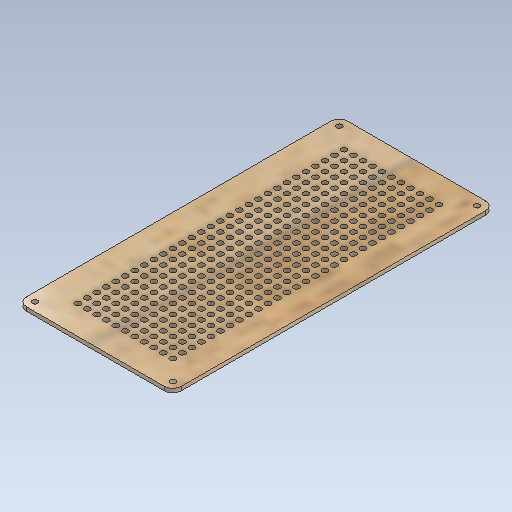
# Autodesk Inventor part: ロボット回転_回路ボード1
Saved by Autodesk Inventor 2020.3 (Build 243373000, 373)
## iProperties
Created: 2020-07-06
Part Number: ロボット回転_回路ボード1
Material: 木材 (カエデ材)
Document SubType Name: Modeling
Designer: totot
Mass: 15.376 g
Surface Area: 300.242 cm^2
Volume: 22.9492 cm^3
Density: 0.67 g/cm^3
Appearance: ナチュラル カエデ材 - 光沢 濃い着色
Author: totot
Autodesk Inventor part; units mm, degrees
ref_plane "YZ Plane" through (0, 0, 0) normal (1, 0, 0) x (0, 1, 0)
ref_plane "XZ Plane" through (0, 0, 0) normal (0, 1, 0) x (-1, 0, 0)
ref_plane "XY Plane" through (0, 0, 0) normal (0, 0, 1) x (1, 0, 0)
sketch "スケッチ1" plane through (0, 0, 0) normal (0, 1, 0) x (-1, 0, 0)
  line L0 (0, 0) -> (-81.5097, 0)
  line L1 (-81.5097, 0) -> (-81.5097, -169)
  line L2 (-81.5097, -169) -> (0, -169)
  line L3 (0, -169) -> (0, 0)
  dimension "d0" = 169
  dimension "d7" = 81.5097
  constraints: 8 end point, 2 parallel, 1 horizontal, 1 perpendicular
  measures "d0" distance of L1.end L0.end
  measures "d7" distance between parallel lines of L1 L3
extrude "押し出し1" add sketch "スケッチ1" along normal blind 2
sketch "スケッチ2" plane through (0, 2, 0) normal (0, 1, 0) x (1, 0, 0)
  line L0 (4.5, 4.5) -> (77.01, 4.5)
  line L1 (77.01, 4.5) -> (77.01, 164.5)
  line L2 (77.01, 164.5) -> (4.5, 164.5)
  line L3 (4.5, 164.5) -> (4.5, 4.5)
  line L4 (0, 169) -> (0, 0) projected
  line L5 (0, 0) -> (81.5097, 0) projected
  line L6 (81.5097, 0) -> (81.5097, 169) projected
  point P0 (66.5097, 15)
  point P1 (61.5097, 15)
  point P2 (56.5097, 15)
  point P3 (51.5097, 15)
  point P4 (46.5097, 15)
  point P5 (41.5097, 15)
  point P6 (36.5097, 15)
  point P7 (31.5097, 15)
  point P8 (26.5097, 15)
  point P9 (21.5097, 15)
  point P10 (16.5097, 15)
  point P11 (66.5097, 20)
  point P12 (61.5097, 20)
  point P13 (56.5097, 20)
  point P14 (51.5097, 20)
  point P15 (46.5097, 20)
  point P16 (41.5097, 20)
  point P17 (36.5097, 20)
  point P18 (31.5097, 20)
  point P19 (26.5097, 20)
  point P20 (21.5097, 20)
  point P21 (16.5097, 20)
  point P22 (66.5097, 25)
  point P23 (61.5097, 25)
  point P24 (56.5097, 25)
  point P25 (51.5097, 25)
  point P26 (46.5097, 25)
  point P27 (41.5097, 25)
  point P28 (36.5097, 25)
  point P29 (31.5097, 25)
  point P30 (26.5097, 25)
  point P31 (21.5097, 25)
  point P32 (16.5097, 25)
  point P33 (66.5097, 30)
  point P34 (61.5097, 30)
  point P35 (56.5097, 30)
  point P36 (51.5097, 30)
  point P37 (46.5097, 30)
  point P38 (41.5097, 30)
  point P39 (36.5097, 30)
  point P40 (31.5097, 30)
  point P41 (26.5097, 30)
  point P42 (21.5097, 30)
  point P43 (16.5097, 30)
  point P44 (66.5097, 35)
  point P45 (61.5097, 35)
  point P46 (56.5097, 35)
  point P47 (51.5097, 35)
  point P48 (46.5097, 35)
  point P49 (41.5097, 35)
  point P50 (36.5097, 35)
  point P51 (31.5097, 35)
  point P52 (26.5097, 35)
  point P53 (21.5097, 35)
  point P54 (16.5097, 35)
  point P55 (66.5097, 40)
  point P56 (61.5097, 40)
  point P57 (56.5097, 40)
  point P58 (51.5097, 40)
  point P59 (46.5097, 40)
  point P60 (41.5097, 40)
  point P61 (36.5097, 40)
  point P62 (31.5097, 40)
  point P63 (26.5097, 40)
  point P64 (21.5097, 40)
  point P65 (16.5097, 40)
  point P66 (66.5097, 45)
  point P67 (61.5097, 45)
  point P68 (56.5097, 45)
  point P69 (51.5097, 45)
  point P70 (46.5097, 45)
  point P71 (41.5097, 45)
  point P72 (36.5097, 45)
  point P73 (31.5097, 45)
  point P74 (26.5097, 45)
  point P75 (21.5097, 45)
  point P76 (16.5097, 45)
  point P77 (66.5097, 50)
  point P78 (61.5097, 50)
  point P79 (56.5097, 50)
  point P80 (51.5097, 50)
  point P81 (46.5097, 50)
  point P82 (41.5097, 50)
  point P83 (36.5097, 50)
  point P84 (31.5097, 50)
  point P85 (26.5097, 50)
  point P86 (21.5097, 50)
  point P87 (16.5097, 50)
  point P88 (66.5097, 55)
  point P89 (61.5097, 55)
  point P90 (56.5097, 55)
  point P91 (51.5097, 55)
  point P92 (46.5097, 55)
  point P93 (41.5097, 55)
  point P94 (36.5097, 55)
  point P95 (31.5097, 55)
  point P96 (26.5097, 55)
  point P97 (21.5097, 55)
  point P98 (16.5097, 55)
  point P99 (66.5097, 60)
  point P100 (61.5097, 60)
  point P101 (56.5097, 60)
  point P102 (51.5097, 60)
  point P103 (46.5097, 60)
  point P104 (41.5097, 60)
  point P105 (36.5097, 60)
  point P106 (31.5097, 60)
  point P107 (26.5097, 60)
  point P108 (21.5097, 60)
  point P109 (16.5097, 60)
  point P110 (66.5097, 65)
  point P111 (61.5097, 65)
  point P112 (56.5097, 65)
  point P113 (51.5097, 65)
  point P114 (46.5097, 65)
  point P115 (41.5097, 65)
  point P116 (36.5097, 65)
  point P117 (31.5097, 65)
  point P118 (26.5097, 65)
  point P119 (21.5097, 65)
  point P120 (16.5097, 65)
  point P121 (66.5097, 70)
  point P122 (61.5097, 70)
  point P123 (56.5097, 70)
  point P124 (51.5097, 70)
  point P125 (46.5097, 70)
  point P126 (41.5097, 70)
  point P127 (36.5097, 70)
  point P128 (31.5097, 70)
  point P129 (26.5097, 70)
  point P130 (21.5097, 70)
  point P131 (16.5097, 70)
  point P132 (66.5097, 75)
  point P133 (61.5097, 75)
  point P134 (56.5097, 75)
  point P135 (51.5097, 75)
  point P136 (46.5097, 75)
  point P137 (41.5097, 75)
  point P138 (36.5097, 75)
  point P139 (31.5097, 75)
  point P140 (26.5097, 75)
  point P141 (21.5097, 75)
  point P142 (16.5097, 75)
  point P143 (66.5097, 80)
  point P144 (61.5097, 80)
  point P145 (56.5097, 80)
  point P146 (51.5097, 80)
  point P147 (46.5097, 80)
  point P148 (41.5097, 80)
  point P149 (36.5097, 80)
  point P150 (31.5097, 80)
  point P151 (26.5097, 80)
  point P152 (21.5097, 80)
  point P153 (16.5097, 80)
  point P154 (66.5097, 85)
  point P155 (61.5097, 85)
  point P156 (56.5097, 85)
  point P157 (51.5097, 85)
  point P158 (46.5097, 85)
  point P159 (41.5097, 85)
  point P160 (36.5097, 85)
  point P161 (31.5097, 85)
  point P162 (26.5097, 85)
  point P163 (21.5097, 85)
  point P164 (16.5097, 85)
  point P165 (66.5097, 90)
  point P166 (61.5097, 90)
  point P167 (56.5097, 90)
  point P168 (51.5097, 90)
  point P169 (46.5097, 90)
  point P170 (41.5097, 90)
  point P171 (36.5097, 90)
  point P172 (31.5097, 90)
  point P173 (26.5097, 90)
  point P174 (21.5097, 90)
  point P175 (16.5097, 90)
  point P176 (66.5097, 95)
  point P177 (61.5097, 95)
  point P178 (56.5097, 95)
  point P179 (51.5097, 95)
  point P180 (46.5097, 95)
  point P181 (41.5097, 95)
  point P182 (36.5097, 95)
  point P183 (31.5097, 95)
  point P184 (26.5097, 95)
  point P185 (21.5097, 95)
  point P186 (16.5097, 95)
  point P187 (66.5097, 100)
  point P188 (61.5097, 100)
  point P189 (56.5097, 100)
  point P190 (51.5097, 100)
  point P191 (46.5097, 100)
  point P192 (41.5097, 100)
  point P193 (36.5097, 100)
  point P194 (31.5097, 100)
  point P195 (26.5097, 100)
  point P196 (21.5097, 100)
  point P197 (16.5097, 100)
  point P198 (66.5097, 105)
  point P199 (61.5097, 105)
  dimension "d3" = 160
  dimension "d4" = 4.5
  dimension "d5" = 4.5
  dimension "d6" = 72.51
  dimension "d8" = 15
  dimension "d9" = 15
  dimension "d12" = 5
  dimension "d15" = 5
  dimension "d28" = 5
  dimension "d31" = 5
  constraints: 8 end point, 4 coincident, 3 horizontal, 2 parallel, 2 vertical, 1 perpendicular, 328 other
  measures "d3" distance of L1.end L0.end
  measures "d4" distance between parallel lines of L3 L4
  measures "d5" distance between parallel lines of L5 L0
  measures "d6" distance between parallel lines of L3 L1
  measures "d8" distance from line of point (66.51, 15) L5
  measures "d9" distance from line of point (66.51, 15) L6
  measures "d12" distance of point (66.51, 15) point (61.51, 15)
  measures "d15" distance of point (66.51, 15) point (66.51, 20)
  measures "d28" distance of point (66.51, 145) point (66.51, 150)
  measures "d31" distance of point (66.51, 145) point (61.51, 145)
hole "穴1" at (4.5, 2, -4.5) at (4.5, 2, -164.5) at (77.01, 2, -164.5) at (77.01, 2, -4.5) at (66.5097, 2, -15) at (61.5097, 2, -15) at (56.5097, 2, -15) at (51.5097, 2, -15) at (46.5097, 2, -15) at (41.5097, 2, -15) at (36.5097, 2, -15) at (31.5097, 2, -15) at (26.5097, 2, -15) at (21.5097, 2, -15) at (16.5097, 2, -15) at (66.5097, 2, -20) at (61.5097, 2, -20) at (56.5097, 2, -20) at (51.5097, 2, -20) at (46.5097, 2, -20) at (41.5097, 2, -20) at (36.5097, 2, -20) at (31.5097, 2, -20) at (26.5097, 2, -20) at (21.5097, 2, -20) at (16.5097, 2, -20) at (66.5097, 2, -25) at (61.5097, 2, -25) at (56.5097, 2, -25) at (51.5097, 2, -25) at (46.5097, 2, -25) at (41.5097, 2, -25) at (36.5097, 2, -25) at (31.5097, 2, -25) at (26.5097, 2, -25) at (21.5097, 2, -25) at (16.5097, 2, -25) at (66.5097, 2, -30) at (61.5097, 2, -30) at (56.5097, 2, -30) at (51.5097, 2, -30) at (46.5097, 2, -30) at (41.5097, 2, -30) at (36.5097, 2, -30) at (31.5097, 2, -30) at (26.5097, 2, -30) at (21.5097, 2, -30) at (16.5097, 2, -30) at (66.5097, 2, -35) at (61.5097, 2, -35) direction (0, -1, 0) diameter 3 end through all and at (56.5097, 2, -35) (51.5097, 2, -35) (46.5097, 2, -35) (41.5097, 2, -35) (36.5097, 2, -35) (31.5097, 2, -35) (26.5097, 2, -35) (21.5097, 2, -35) (16.5097, 2, -35) (66.5097, 2, -40) (61.5097, 2, -40) (56.5097, 2, -40) (51.5097, 2, -40) (46.5097, 2, -40) (41.5097, 2, -40) (36.5097, 2, -40) (31.5097, 2, -40) (26.5097, 2, -40) (21.5097, 2, -40) (16.5097, 2, -40) (66.5097, 2, -45) (61.5097, 2, -45) (56.5097, 2, -45) (51.5097, 2, -45) (46.5097, 2, -45) (41.5097, 2, -45) (36.5097, 2, -45) (31.5097, 2, -45) (26.5097, 2, -45) (21.5097, 2, -45) (16.5097, 2, -45) (66.5097, 2, -50) (61.5097, 2, -50) (56.5097, 2, -50) (51.5097, 2, -50) (46.5097, 2, -50) (41.5097, 2, -50) (36.5097, 2, -50) (31.5097, 2, -50) (26.5097, 2, -50) (21.5097, 2, -50) (16.5097, 2, -50) (66.5097, 2, -55) (61.5097, 2, -55) (56.5097, 2, -55) (51.5097, 2, -55) (46.5097, 2, -55) (41.5097, 2, -55) (36.5097, 2, -55) (31.5097, 2, -55) (26.5097, 2, -55) (21.5097, 2, -55) (16.5097, 2, -55) (66.5097, 2, -60) (61.5097, 2, -60) (56.5097, 2, -60) (51.5097, 2, -60) (46.5097, 2, -60) (41.5097, 2, -60) (36.5097, 2, -60) (31.5097, 2, -60) (26.5097, 2, -60) (21.5097, 2, -60) (16.5097, 2, -60) (66.5097, 2, -65) (61.5097, 2, -65) (56.5097, 2, -65) (51.5097, 2, -65) (46.5097, 2, -65) (41.5097, 2, -65) (36.5097, 2, -65) (31.5097, 2, -65) (26.5097, 2, -65) (21.5097, 2, -65) (16.5097, 2, -65) (66.5097, 2, -70) (61.5097, 2, -70) (56.5097, 2, -70) (51.5097, 2, -70) (46.5097, 2, -70) (41.5097, 2, -70) (36.5097, 2, -70) (31.5097, 2, -70) (26.5097, 2, -70) (21.5097, 2, -70) (16.5097, 2, -70) (66.5097, 2, -75) (61.5097, 2, -75) (56.5097, 2, -75) (51.5097, 2, -75) (46.5097, 2, -75) (41.5097, 2, -75) (36.5097, 2, -75) (31.5097, 2, -75) (26.5097, 2, -75) (21.5097, 2, -75) (16.5097, 2, -75) (66.5097, 2, -80) (61.5097, 2, -80) (56.5097, 2, -80) (51.5097, 2, -80) (46.5097, 2, -80) (41.5097, 2, -80) (36.5097, 2, -80) (31.5097, 2, -80) (26.5097, 2, -80) (21.5097, 2, -80) (16.5097, 2, -80) (66.5097, 2, -85) (61.5097, 2, -85) (56.5097, 2, -85) (51.5097, 2, -85) (46.5097, 2, -85) (41.5097, 2, -85) (36.5097, 2, -85) (31.5097, 2, -85) (26.5097, 2, -85) (21.5097, 2, -85) (16.5097, 2, -85) (66.5097, 2, -90) (61.5097, 2, -90) (56.5097, 2, -90) (51.5097, 2, -90) (46.5097, 2, -90) (41.5097, 2, -90) (36.5097, 2, -90) (31.5097, 2, -90) (26.5097, 2, -90) (21.5097, 2, -90) (16.5097, 2, -90) (66.5097, 2, -95) (61.5097, 2, -95) (56.5097, 2, -95) (51.5097, 2, -95) (46.5097, 2, -95) (41.5097, 2, -95) (36.5097, 2, -95) (31.5097, 2, -95) (26.5097, 2, -95) (21.5097, 2, -95) (16.5097, 2, -95) (66.5097, 2, -100) (61.5097, 2, -100) (56.5097, 2, -100) (51.5097, 2, -100) (46.5097, 2, -100) (41.5097, 2, -100) (36.5097, 2, -100) (31.5097, 2, -100) (26.5097, 2, -100) (21.5097, 2, -100) (16.5097, 2, -100) (66.5097, 2, -105) (61.5097, 2, -105) (56.5097, 2, -105) (51.5097, 2, -105) (46.5097, 2, -105) (41.5097, 2, -105) (36.5097, 2, -105) (31.5097, 2, -105) (26.5097, 2, -105) (21.5097, 2, -105) (16.5097, 2, -105) (66.5097, 2, -110) (61.5097, 2, -110) (56.5097, 2, -110) (51.5097, 2, -110) (46.5097, 2, -110) (41.5097, 2, -110) (36.5097, 2, -110) (31.5097, 2, -110) (26.5097, 2, -110) (21.5097, 2, -110) (16.5097, 2, -110) (66.5097, 2, -115) (61.5097, 2, -115) (56.5097, 2, -115) (51.5097, 2, -115) (46.5097, 2, -115) (41.5097, 2, -115) (36.5097, 2, -115) (31.5097, 2, -115) (26.5097, 2, -115) (21.5097, 2, -115) (16.5097, 2, -115) (66.5097, 2, -120) (61.5097, 2, -120) (56.5097, 2, -120) (51.5097, 2, -120) (46.5097, 2, -120) (41.5097, 2, -120) (36.5097, 2, -120) (31.5097, 2, -120) (26.5097, 2, -120) (21.5097, 2, -120) (16.5097, 2, -120) (66.5097, 2, -125) (61.5097, 2, -125) (56.5097, 2, -125) (51.5097, 2, -125) (46.5097, 2, -125) (41.5097, 2, -125) (36.5097, 2, -125) (31.5097, 2, -125) (26.5097, 2, -125) (21.5097, 2, -125) (16.5097, 2, -125) (66.5097, 2, -130) (61.5097, 2, -130) (56.5097, 2, -130) (51.5097, 2, -130) (46.5097, 2, -130) (41.5097, 2, -130) (36.5097, 2, -130) (31.5097, 2, -130) (26.5097, 2, -130) (21.5097, 2, -130) (16.5097, 2, -130) (66.5097, 2, -135) (61.5097, 2, -135) (56.5097, 2, -135) (51.5097, 2, -135) (46.5097, 2, -135) (41.5097, 2, -135) (36.5097, 2, -135) (31.5097, 2, -135) (26.5097, 2, -135) (21.5097, 2, -135) (16.5097, 2, -135) (66.5097, 2, -140) (61.5097, 2, -140) (56.5097, 2, -140) (51.5097, 2, -140) (46.5097, 2, -140) (41.5097, 2, -140) (36.5097, 2, -140) (31.5097, 2, -140) (26.5097, 2, -140) (21.5097, 2, -140) (16.5097, 2, -140) (66.5097, 2, -145) (61.5097, 2, -145) (56.5097, 2, -145) (51.5097, 2, -145) (46.5097, 2, -145) (41.5097, 2, -145) (36.5097, 2, -145) (31.5097, 2, -145) (26.5097, 2, -145) (21.5097, 2, -145) (16.5097, 2, -145) (16.5097, 2, -150) (16.5097, 2, -155) (21.5097, 2, -155) (21.5097, 2, -150) (26.5097, 2, -155) (26.5097, 2, -150) (31.5097, 2, -150) (36.5097, 2, -150) (41.5097, 2, -150) (46.5097, 2, -150) (31.5097, 2, -155) (36.5097, 2, -155) (51.5097, 2, -150) (56.5097, 2, -150) (56.5097, 2, -155) (51.5097, 2, -155) (46.5097, 2, -155) (41.5097, 2, -155) (66.5097, 2, -150) (61.5097, 2, -150) (66.5097, 2, -155) (61.5097, 2, -155)
fillet "フィレット1" radius 4.5 4 edges at (81.5097, 1, 0) (0, 1, 0) (81.5097, 1, -169) (0, 1, -169)
equation "\"d4\" = d5"
